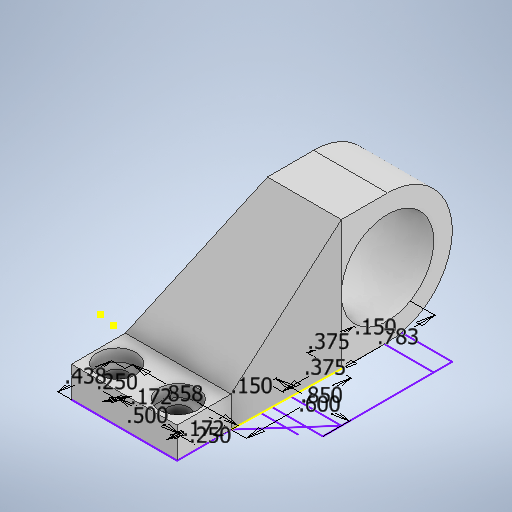
# Autodesk Inventor part: Air Tank Mount 2
Saved by Autodesk Inventor 2025.1 (Build 291241020, 241B)
## iProperties
Created: 2025-01-07
Part Number: Air Tank Mount 2
Material: Generic
Document SubType Name: Modeling
Designer: AtuStem
Density: 1 g/cm^3
Appearance: Default
Author: AtuStem
Autodesk Inventor part; units mm, degrees
ref_plane "YZ Plane" through (0, 0, 0) normal (1, 0, 0) x (0, 1, 0)
ref_plane "XZ Plane" through (0, 0, 0) normal (0, 1, 0) x (-1, 0, 0)
ref_plane "XY Plane" through (0, 0, 0) normal (0, 0, 1) x (1, 0, 0)
sketch "Sketch1" plane through (0, 0, 0) normal (0, 1, 0) x (-1, 0, 0)
  circle A0 centre (-13.5035, 12.9456) radius 2.1844
  circle A1 centre (-26.2035, 12.9456) radius 2.1844
  line L0 (-30.2421, 5.5256) -> (-22.1649, 5.5256)
  line L1 (-17.5421, 5.5256) -> (-9.4649, 5.5256)
  line L2 (-8.9569, 17.7081) -> (-30.7501, 17.7081)
  line L3 (-8.9569, 17.7081) -> (-30.7501, 17.7081)
  line L4 (-30.7501, 17.7081) -> (-30.7501, 6.5956)
  line L5 (-30.7501, 6.5956) -> (-8.9569, 6.5956)
  line L6 (-8.9569, 6.5956) -> (-8.9569, 17.7081)
  line L7 (-26.2035, 6.5956) -> (-26.2035, -14.9944)
  line L8 (-26.2035, -14.9944) -> (-26.2035, -34.8699)
  line L9 (-26.2035, -14.9944) -> (-26.2035, -5.4694)
  line L10 (-26.2035, -14.9944) -> (-26.2035, -24.5194)
  line L11 (-26.2035, -24.5194) -> (-26.2035, -28.3294)
  line L12 (-26.2035, -5.4694) -> (-26.2035, -1.6594)
  line L13 (-26.2035, -1.6594) -> (-41.4435, -1.6594)
  line L14 (-26.2035, -28.3294) -> (-41.4435, -28.3294)
  line L15 (-41.4435, -28.3294) -> (-41.4435, -1.6594)
  line L16 (-26.2035, -24.5194) -> (-41.4435, -24.5194)
  line L17 (-26.2035, -5.4694) -> (-41.4435, -5.4694)
  line L18 (-8.9569, 6.5956) -> (-26.2035, -5.4694)
  line L19 (-17.5802, 0.5631) -> (-38.5645, 0.5631)
  line L20 (-30.7501, 6.5956) -> (-41.4435, -5.4694)
  point P0 (0, 0)
  point P1 (-26.2035, 0.5631)
  dimension "d0" = 4.3688
  dimension "d1" = 4.3688
  dimension "d2" = 12.7
  dimension "d3" = 11.1125
  dimension "d4" = 21.7932
  dimension "d5" = 6.35
  dimension "d6" = 6.35
  dimension "d9" = 21.59
  dimension "d10" = 19.8755
  dimension "d11" = 9.525
  dimension "d12" = 9.525
  dimension "d13" = 3.81
  dimension "d14" = 3.81
  dimension "d15" = 15.24
  constraints: 42 end point, 7 point on line, 5 perpendicular, 4 horizontal, 2 centre point, 2 parallel, 1 midpoint, 1 vertical
  measures "d0" diameter of A0
  measures "d1" diameter of A1
  measures "d2" distance of A0.centre A1.centre
  measures "d3" distance of L5.end L2.start
  measures "d4" distance of L4.end L5.end
  measures "d5" distance from line of L5 A0.centre
  measures "d6" distance from line of L5 A1.centre
  measures "d9" distance of L7.start L7.end
  measures "d10" distance of L7.end L8.end
  measures "d11" distance of L9.end L7.end
  measures "d12" distance of L10.end L7.end
  measures "d13" distance of L11.end L10.end
  measures "d14" distance of L9.end L12.end
  measures "d15" distance of L12.end L13.end
extrude "Extrusion11" add sketch "Sketch1" along normal blind 3.81 contours L6 L5 L4 L2
sketch "Sketch11" plane through (0, 3.81, 0) normal (0, 1, 0) x (1, 0, 0)
  circle A0 centre (13.5035, -12.9456) radius 2.1844 projected
  circle A1 centre (13.5035, -12.9456) radius 3.9624
  circle A2 centre (26.2035, -12.9456) radius 2.1844 projected
  circle A3 centre (26.2035, -12.9456) radius 3.9624
  line L0 (30.7501, -6.5956) -> (8.9569, -6.5956) projected
  line L1 (30.7501, -17.7081) -> (30.7501, -6.5956) projected
  line L2 (8.9569, -6.5956) -> (30.7501, -6.5956)
  line L3 (30.7501, -6.5956) -> (30.7501, -17.7081)
  line L4 (30.7501, -17.7081) -> (8.9569, -17.7081)
  line L5 (8.9569, -17.7081) -> (8.9569, -6.5956)
  point P0 (0, 0)
  dimension "d48" = 7.9248
  dimension "d49" = 7.9248
  constraints: 8 end point, 2 centre point, 2 coincident, 2 parallel, 1 horizontal, 1 perpendicular
  measures "d48" diameter of A1
  measures "d49" diameter of A3
extrude "Extrusion12" add sketch "Sketch11" along normal blind 2.54 contours L1 L4 L5 L0
extrude "Extrusion13" add sketch "Sketch1" along normal blind 6.35 contours L18 L19 L7 L5 | L5 L7 L19 L20 | L19 L7 L13 L20 | L18 L7 L19 | L13 L7 L17 L20
extrude "Extrusion15" add sketch "Sketch1" along normal blind 36.83 contours L7 L8 L16 L15 L17 | L16 L8 L14 L15
sketch "Sketch13" plane through (41.4435, 0, -5.4694) normal (1, 0, 0) x (0, 0, -1)
  line L0 (0, 0) -> (0, 6.35) projected
  line L1 (22.86, 0) -> (22.86, 36.83) projected
  line L2 (0, 0) -> (22.86, 0)
  line L3 (22.86, 0) -> (22.86, 10.16)
  line L4 (22.86, 10.16) -> (0, 10.16)
  line L5 (0, 10.16) -> (0, 0)
  line L6 (0, 10.16) -> (9.525, 10.16)
  line L7 (9.525, 10.16) -> (9.525, 23.495)
  line L8 (9.525, 23.495) -> (0, 23.495)
  line L9 (0, 23.495) -> (0, 10.16)
  circle A0 centre (9.525, 23.495) radius 9.525
  circle A1 centre (9.525, 23.495) radius 13.335
  line L10 (0, 36.83) -> (22.86, 36.83) projected
  line L11 (0, 36.83) -> (22.86, 36.83)
  line L12 (22.86, 36.83) -> (22.86, 10.16)
  line L13 (22.86, 10.16) -> (0, 10.16)
  line L14 (0, 10.16) -> (0, 36.83)
  point P0 (-5.4694, 0)
  point P1 (9.525, 36.83)
  point P2 (22.86, 23.495)
  point P3 (9.525, 10.16)
  dimension "d62" = 10.16
  dimension "d63" = 9.525
  dimension "d64" = 13.335
  dimension "d65" = 19.05
  dimension "d66" = 26.67
  dimension "d67" = 36.83
  constraints: 24 end point, 6 parallel, 3 horizontal, 3 perpendicular, 2 centre point, 2 coincident, 1 point on line
  measures "d62" distance of L4.end L0.start
  measures "d63" distance of L7.end L8.end
  measures "d64" distance of L6.end L7.end
  measures "d65" diameter of A0
  measures "d66" diameter of A1
  measures "d67" distance of L1.start L1.end
extrude "Extrusion16" cut sketch "Sketch13" against normal up to surface (15.24 mm away) contours L0 L5 L4 L1 L2 | L4 A1 L1 | A1 L10 L1 | A0 L8 L7 | L7 L8 A0
sketch "Sketch20" plane through (0, 6.35, 0) normal (0, 1, 0) x (1, 0, 0)
  line L0 (26.2035, 5.4694) -> (8.9569, -6.5956) projected
  line L1 (30.7501, -6.5956) -> (41.4435, 5.4694) projected
  line L2 (8.9569, -6.5956) -> (30.7501, -6.5956)
  line L3 (30.7501, -6.5956) -> (41.4435, 5.4694)
  line L4 (26.2035, 14.9944) -> (26.2035, 5.4694) projected
  line L5 (41.4435, 5.4694) -> (26.2035, 5.4694)
  line L6 (26.2035, 5.4694) -> (8.9569, -6.5956)
  point P0 (0, 0)
  constraints: 8 end point, 1 collinear, 1 horizontal, 1 parallel
extrude "Extrusion17" add sketch "Sketch20" along normal up to surface (30.48 mm away)
sketch "Sketch21" plane through (30.7501, 0, 17.7081) normal (1, 0, 0) x (0, 0, -1)
  line L0 (11.1125, 0) -> (11.1125, 6.35) projected
  line L1 (23.1775, 36.83) -> (32.7025, 36.83) projected
  line L2 (11.1125, 6.35) -> (23.1775, 36.83)
  line L3 (23.1775, 36.83) -> (11.1125, 36.83) projected
  line L4 (11.1125, 6.35) -> (11.1125, 36.83)
  line L5 (11.1125, 36.83) -> (23.1775, 36.83)
  point P0 (17.7081, 0)
  constraints: 6 end point, 1 vertical
extrude "Extrusion18" cut sketch "Sketch21" against normal up to surface surface through (26.2035, 0, -5.4694) normal (-0.5732193, 0, -0.819402)
extrude "Extrusion19" cut sketch "Sketch21" against normal up to surface surface through (30.7501, 0, 6.5956) normal (0.7483647, 0, 0.6632875)
sketch "Sketch22" plane through (30.7501, 0, 17.7081) normal (1, 0, 0) x (0, 0, -1)
  line L0 (11.1125, 0) -> (23.1775, 0) projected
  line L1 (23.1775, 0) -> (23.1775, 10.16) projected
  line L2 (11.1125, 0) -> (23.1775, 10.16)
  line L3 (11.1125, 0) -> (23.1775, 0)
  line L4 (23.1775, 10.16) -> (23.1775, 0)
  point P0 (17.7081, 0)
  constraints: 6 end point, 1 collinear, 1 perpendicular
extrude "Extrusion20" cut sketch "Sketch22" against normal up to surface (21.7932 mm away)
extrude "Extrusion21" cut sketch "Sketch22" along normal blind 25.4
fillet "Fillet1" [suppressed]
fillet "Fillet2" [suppressed]
fillet "Fillet3" [suppressed]
fillet "Fillet4" [suppressed]
sketch "Sketch23" plane through (8.9569, 0, 6.5956) normal (0, -0.7649112, -0.6441357) x (1, 0, 0)
  line L0 (17.2466, -15.7731) -> (0, 0) projected
  line L1 (17.2466, -15.7731) -> (32.4866, -15.7731) projected
  line L2 (21.7932, 0) -> (32.4866, -15.7731) projected
  line L3 (0, 0) -> (21.7932, 0) projected
  point P0 (-8.9569, -5.045)
equation "\"d68\" = d65"
body "Solid2"
